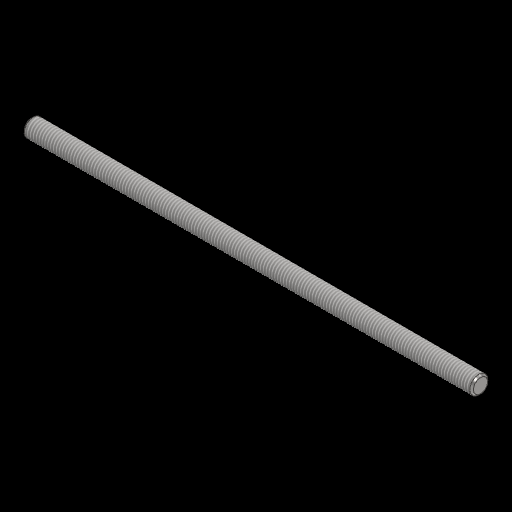
# Autodesk Inventor part: ThreadedRod-M4x125
Saved by Autodesk Inventor 2024 (Build 280153000, 153)
## iProperties
Created: 2023-06-30
Part Number: ThreadedRod-M4x125
Material: Edelstahl
Document SubType Name: Modeling
Designer: buchmannmartin
Density: 8 g/cm^3
Appearance: Halbpoliert
Description: Gewindestange M5; 125mm lang
Mass: 19.6056 g
Surface Area: 19.9291 cm^2
Volume: 2.4507 cm^3
Author: buchmannmartin
Autodesk Inventor part; units mm, degrees
ref_plane "YZ Plane" through (0, 0, 0) normal (1, 0, 0) x (0, 1, 0)
ref_plane "XZ Plane" through (0, 0, 0) normal (0, 1, 0) x (-1, 0, 0)
ref_plane "XY Plane" through (0, 0, 0) normal (0, 0, 1) x (1, 0, 0)
sketch "Skizze1" plane through (0, 0, 0) normal (0, 0, 1) x (1, 0, 0)
  line L0 (0, 0) -> (125, 0)
  line L1 (125, 0) -> (125, 2.5)
  line L2 (125, 2.5) -> (0, 2.5)
  line L3 (0, 2.5) -> (0, 0)
  dimension "d0" = 5
  dimension "d1" = 125
  constraints: 8 end point, 2 parallel, 1 horizontal, 1 perpendicular
  measures "d0" diameter of L2 L0
  measures "d1" distance of L0.start L0.end
revolve "Umdrehung1" add sketch "Skizze1" angle 360 about axis through (0, 0, 0) along (1, 0, 0)
chamfer "Fasen1" distance 0.5 angle 45 2 edges at (0, -2.5, 0) (125, -2.5, 0)
thread "Gewinde1" size "M5x0.8" class "6g" standard "ANSI Metric M Profile" full length
